Autodesk Inventor part; units mm, degrees
(part 2 of 3)
  arc A299 (127, -169.8625) -> (130.175, -173.0375) centre (130.175, -169.8625) ccw
  arc A300 (132.08, -138.7475) -> (127, -141.2875) centre (130.175, -141.2875) ccw
  arc A301 (136.525, -119.0625) -> (134.62, -124.7775) centre (136.525, -122.2375) ccw
  line L312 (172.72, -153.3525) -> (134.62, -124.7775)
  line L313 (136.525, -119.0625) -> (174.625, -119.0625)
  line L314 (177.8, -122.2375) -> (177.8, -150.8125)
  line L315 (170.18, -167.3225) -> (132.08, -138.7475)
  line L316 (130.175, -173.0375) -> (168.275, -173.0375)
  arc A302 (168.275, -173.0375) -> (170.18, -167.3225) centre (168.275, -169.8625) ccw
  line L317 (-187.4223, -179.3875) -> (-42.9584, -179.3875) construction
  line L318 (-189.0098, -179.3875) -> (-44.5459, -179.3875) construction
  arc A303 (106.68, -124.7775) -> (104.775, -119.0625) centre (104.775, -122.2375) ccw
  line L319 (63.5, -122.2375) -> (63.5, -150.8125)
  arc A304 (63.5, -150.8125) -> (68.58, -153.3525) centre (66.675, -150.8125) ccw
  line L320 (68.58, -153.3525) -> (106.68, -124.7775)
  arc A305 (114.3, -141.2875) -> (109.22, -138.7475) centre (111.125, -141.2875) ccw
  line L321 (71.12, -167.3225) -> (109.22, -138.7475)
  line L322 (111.125, -173.0375) -> (73.025, -173.0375)
  line L323 (120.65, 393.4968) -> (120.65, 317.2968) construction
  line L324 (114.3, -141.2875) -> (114.3, -169.8625)
  arc A306 (111.125, -173.0375) -> (114.3, -169.8625) centre (111.125, -169.8625) ccw
  arc A307 (114.3, -188.9125) -> (111.125, -185.7375) centre (111.125, -188.9125) ccw
  line L325 (114.3, -217.4875) -> (114.3, -188.9125)
  line L326 (111.125, -185.7375) -> (73.025, -185.7375)
  arc A308 (73.025, -185.7375) -> (71.12, -191.4525) centre (73.025, -188.9125) ccw
  line L327 (71.12, -191.4525) -> (109.22, -220.0275)
  arc A309 (68.58, -205.4225) -> (63.5, -207.9625) centre (66.675, -207.9625) ccw
  line L328 (68.58, -205.4225) -> (106.68, -233.9975)
  line L329 (104.775, -239.7125) -> (66.675, -239.7125)
  line L330 (63.5, -236.5375) -> (63.5, -207.9625)
  arc A310 (63.5, -236.5375) -> (66.675, -239.7125) centre (66.675, -236.5375) ccw
  arc A311 (71.12, -167.3225) -> (73.025, -173.0375) centre (73.025, -169.8625) ccw
  line L331 (127, -217.4875) -> (127, -188.9125)
  arc A312 (104.775, -239.7125) -> (106.68, -233.9975) centre (104.775, -236.5375) ccw
  arc A313 (109.22, -220.0275) -> (114.3, -217.4875) centre (111.125, -217.4875) ccw
  arc A314 (177.8, -122.2375) -> (174.625, -119.0625) centre (174.625, -122.2375) ccw
  arc A315 (172.72, -153.3525) -> (177.8, -150.8125) centre (174.625, -150.8125) ccw
  arc A316 (198.12, -167.3225) -> (200.025, -173.0375) centre (200.025, -169.8625) ccw
  arc A317 (190.5, -150.8125) -> (195.58, -153.3525) centre (193.675, -150.8125) ccw
  line L332 (190.5, -122.2375) -> (190.5, -150.8125)
  arc A318 (193.675, -119.0625) -> (190.5, -122.2375) centre (193.675, -122.2375) ccw
  arc A319 (130.175, -185.7375) -> (127, -188.9125) centre (130.175, -188.9125) ccw
  arc A320 (127, -217.4875) -> (132.08, -220.0275) centre (130.175, -217.4875) ccw
  line L333 (130.175, -185.7375) -> (168.275, -185.7375)
  line L334 (177.8, -236.5375) -> (177.8, -207.9625)
  arc A321 (170.18, -191.4525) -> (168.275, -185.7375) centre (168.275, -188.9125) ccw
  line L335 (195.58, -153.3525) -> (233.68, -124.7775)
  line L336 (231.775, -119.0625) -> (193.675, -119.0625)
  arc A322 (241.3, -141.2875) -> (236.22, -138.7475) centre (238.125, -141.2875) ccw
  line L337 (198.12, -167.3225) -> (236.22, -138.7475)
  arc A323 (241.3, -188.9125) -> (238.125, -185.7375) centre (238.125, -188.9125) ccw
  arc A324 (238.125, -173.0375) -> (241.3, -169.8625) centre (238.125, -169.8625) ccw
  arc A325 (236.22, -220.0275) -> (241.3, -217.4875) centre (238.125, -217.4875) ccw
  arc A326 (231.775, -239.7125) -> (233.68, -233.9975) centre (231.775, -236.5375) ccw
  line L338 (170.18, -191.4525) -> (132.08, -220.0275)
  arc A327 (177.8, -207.9625) -> (172.72, -205.4225) centre (174.625, -207.9625) ccw
  arc A328 (174.625, -239.7125) -> (177.8, -236.5375) centre (174.625, -236.5375) ccw
  line L339 (136.525, -239.7125) -> (174.625, -239.7125)
  arc A329 (134.62, -233.9975) -> (136.525, -239.7125) centre (136.525, -236.5375) ccw
  line L340 (172.72, -205.4225) -> (134.62, -233.9975)
  line L341 (241.3, -141.2875) -> (241.3, -169.8625)
  arc A330 (233.68, -124.7775) -> (231.775, -119.0625) centre (231.775, -122.2375) ccw
  line L342 (238.125, -173.0375) -> (200.025, -173.0375)
  line L343 (241.3, -217.4875) -> (241.3, -188.9125)
  line L344 (238.125, -185.7375) -> (200.025, -185.7375)
  arc A331 (200.025, -185.7375) -> (198.12, -191.4525) centre (200.025, -188.9125) ccw
  line L345 (198.12, -191.4525) -> (236.22, -220.0275)
  arc A332 (195.58, -205.4225) -> (190.5, -207.9625) centre (193.675, -207.9625) ccw
  line L346 (195.58, -205.4225) -> (233.68, -233.9975)
  line L347 (231.775, -239.7125) -> (193.675, -239.7125)
  line L348 (190.5, -236.5375) -> (190.5, -207.9625)
  arc A333 (190.5, -236.5375) -> (193.675, -239.7125) centre (193.675, -236.5375) ccw
  arc A334 (168.275, -306.3875) -> (170.18, -300.6725) centre (168.275, -303.2125) ccw
  line L349 (127, -274.6375) -> (127, -303.2125)
  line L350 (120.65, 395.0843) -> (120.65, 318.8843) construction
  line L351 (170.18, -300.6725) -> (132.08, -272.0975)
  arc A335 (132.08, -272.0975) -> (127, -274.6375) centre (130.175, -274.6375) ccw
  arc A336 (172.72, -286.7025) -> (177.8, -284.1625) centre (174.625, -284.1625) ccw
  line L352 (172.72, -286.7025) -> (134.62, -258.1275)
  line L353 (136.525, -252.4125) -> (174.625, -252.4125)
  line L354 (177.8, -255.5875) -> (177.8, -284.1625)
  arc A337 (177.8, -255.5875) -> (174.625, -252.4125) centre (174.625, -255.5875) ccw
  arc A338 (231.775, -373.0625) -> (233.68, -367.3475) centre (231.775, -369.8875) ccw
  arc A339 (45.72, -286.7025) -> (50.8, -284.1625) centre (47.625, -284.1625) ccw
  arc A340 (50.8, -255.5875) -> (47.625, -252.4125) centre (47.625, -255.5875) ccw
  arc A341 (66.675, -252.4125) -> (63.5, -255.5875) centre (66.675, -255.5875) ccw
  line L355 (63.5, -255.5875) -> (63.5, -284.1625)
  arc A342 (63.5, -284.1625) -> (68.58, -286.7025) centre (66.675, -284.1625) ccw
  line L356 (50.8, -255.5875) -> (50.8, -284.1625)
  line L357 (63.5, -369.8875) -> (63.5, -341.3125)
  arc A343 (63.5, -369.8875) -> (66.675, -373.0625) centre (66.675, -369.8875) ccw
  arc A344 (68.58, -338.7725) -> (63.5, -341.3125) centre (66.675, -341.3125) ccw
  line L358 (104.775, -373.0625) -> (66.675, -373.0625)
  line L359 (68.58, -338.7725) -> (106.68, -367.3475)
  line L360 (71.12, -324.8025) -> (109.22, -353.3775)
  arc A345 (71.12, -300.6725) -> (73.025, -306.3875) centre (73.025, -303.2125) ccw
  arc A346 (73.025, -319.0875) -> (71.12, -324.8025) centre (73.025, -322.2625) ccw
  line L361 (111.125, -306.3875) -> (73.025, -306.3875)
  line L362 (111.125, -319.0875) -> (73.025, -319.0875)
  arc A347 (111.125, -306.3875) -> (114.3, -303.2125) centre (111.125, -303.2125) ccw
  line L363 (104.775, -252.4125) -> (66.675, -252.4125)
  arc A348 (106.68, -258.1275) -> (104.775, -252.4125) centre (104.775, -255.5875) ccw
  line L364 (68.58, -286.7025) -> (106.68, -258.1275)
  line L365 (71.12, -300.6725) -> (109.22, -272.0975)
  arc A349 (114.3, -274.6375) -> (109.22, -272.0975) centre (111.125, -274.6375) ccw
  line L366 (114.3, -274.6375) -> (114.3, -303.2125)
  arc A350 (130.175, -319.0875) -> (127, -322.2625) centre (130.175, -322.2625) ccw
  line L367 (114.3, -350.8375) -> (114.3, -322.2625)
  arc A351 (104.775, -373.0625) -> (106.68, -367.3475) centre (104.775, -369.8875) ccw
  arc A352 (109.22, -353.3775) -> (114.3, -350.8375) centre (111.125, -350.8375) ccw
  line L368 (127, -350.8375) -> (127, -322.2625)
  arc A353 (127, -350.8375) -> (132.08, -353.3775) centre (130.175, -350.8375) ccw
  arc A354 (134.62, -367.3475) -> (136.525, -373.0625) centre (136.525, -369.8875) ccw
  arc A355 (136.525, -252.4125) -> (134.62, -258.1275) centre (136.525, -255.5875) ccw
  arc A356 (170.18, -324.8025) -> (168.275, -319.0875) centre (168.275, -322.2625) ccw
  arc A357 (127, -303.2125) -> (130.175, -306.3875) centre (130.175, -303.2125) ccw
  line L369 (130.175, -319.0875) -> (168.275, -319.0875)
  line L370 (130.175, -306.3875) -> (168.275, -306.3875)
  line L371 (170.18, -324.8025) -> (132.08, -353.3775)
  line L372 (172.72, -338.7725) -> (134.62, -367.3475)
  line L373 (136.525, -373.0625) -> (174.625, -373.0625)
  arc A358 (174.625, -373.0625) -> (177.8, -369.8875) centre (174.625, -369.8875) ccw
  arc A359 (177.8, -341.3125) -> (172.72, -338.7725) centre (174.625, -341.3125) ccw
  line L374 (190.5, -369.8875) -> (190.5, -341.3125)
  line L375 (177.8, -369.8875) -> (177.8, -341.3125)
  arc A360 (190.5, -369.8875) -> (193.675, -373.0625) centre (193.675, -369.8875) ccw
  arc A361 (198.12, -300.6725) -> (200.025, -306.3875) centre (200.025, -303.2125) ccw
  arc A362 (241.3, -274.6375) -> (236.22, -272.0975) centre (238.125, -274.6375) ccw
  line L376 (238.125, -306.3875) -> (200.025, -306.3875)
  line L377 (198.12, -300.6725) -> (236.22, -272.0975)
  arc A363 (233.68, -258.1275) -> (231.775, -252.4125) centre (231.775, -255.5875) ccw
  arc A364 (190.5, -284.1625) -> (195.58, -286.7025) centre (193.675, -284.1625) ccw
  line L378 (195.58, -286.7025) -> (233.68, -258.1275)
  line L379 (231.775, -252.4125) -> (193.675, -252.4125)
  arc A365 (193.675, -252.4125) -> (190.5, -255.5875) centre (193.675, -255.5875) ccw
  line L380 (190.5, -255.5875) -> (190.5, -284.1625)
  line L381 (241.3, -274.6375) -> (241.3, -303.2125)
  arc A366 (238.125, -306.3875) -> (241.3, -303.2125) centre (238.125, -303.2125) ccw
  arc A367 (241.3, -322.2625) -> (238.125, -319.0875) centre (238.125, -322.2625) ccw
  arc A368 (200.025, -319.0875) -> (198.12, -324.8025) centre (200.025, -322.2625) ccw
  line L382 (238.125, -319.0875) -> (200.025, -319.0875)
  arc A369 (236.22, -353.3775) -> (241.3, -350.8375) centre (238.125, -350.8375) ccw
  line L383 (231.775, -373.0625) -> (193.675, -373.0625)
  line L384 (195.58, -338.7725) -> (233.68, -367.3475)
  line L385 (241.3, -350.8375) -> (241.3, -322.2625)
  line L386 (198.12, -324.8025) -> (236.22, -353.3775)
  arc A370 (195.58, -338.7725) -> (190.5, -341.3125) centre (193.675, -341.3125) ccw
  arc A371 (114.3, -322.2625) -> (111.125, -319.0875) centre (111.125, -322.2625) ccw
  line L387 (-142.875, -306.3875) -> (-180.975, -306.3875)
  line L388 (-123.825, -306.3875) -> (-85.725, -306.3875)
  arc A372 (-142.875, -306.3875) -> (-139.7, -303.2125) centre (-142.875, -303.2125) ccw
  line L389 (-185.8348, -312.7375) -> (-41.3709, -312.7375) construction
  line L390 (-189.0098, -312.7375) -> (-44.5459, -312.7375) construction
  line L391 (-127, -350.8375) -> (-127, -322.2625)
  arc A373 (-139.7, -322.2625) -> (-142.875, -319.0875) centre (-142.875, -322.2625) ccw
  line L392 (-187.4223, -312.7375) -> (-42.9584, -312.7375) construction
  line L393 (-187.4223, -312.7375) -> (-42.9584, -312.7375) construction
  arc A374 (-190.5, -369.8875) -> (-187.325, -373.0625) centre (-187.325, -369.8875) ccw
  arc A375 (-117.475, -252.4125) -> (-119.38, -258.1275) centre (-117.475, -255.5875) ccw
  line L394 (-83.82, -300.6725) -> (-121.92, -272.0975)
  line L395 (-81.28, -286.7025) -> (-119.38, -258.1275)
  line L396 (-117.475, -252.4125) -> (-79.375, -252.4125)
  arc A376 (-76.2, -255.5875) -> (-79.375, -252.4125) centre (-79.375, -255.5875) ccw
  line L397 (-76.2, -255.5875) -> (-76.2, -284.1625)
  line L398 (-142.875, -319.0875) -> (-180.975, -319.0875)
  line L399 (-182.88, -324.8025) -> (-144.78, -353.3775)
  arc A377 (-180.975, -319.0875) -> (-182.88, -324.8025) centre (-180.975, -322.2625) ccw
  line L400 (-185.42, -338.7725) -> (-147.32, -367.3475)
  line L401 (-149.225, -373.0625) -> (-187.325, -373.0625)
  line L402 (-190.5, -369.8875) -> (-190.5, -341.3125)
  arc A378 (-185.42, -338.7725) -> (-190.5, -341.3125) centre (-187.325, -341.3125) ccw
  arc A379 (-127, -303.2125) -> (-123.825, -306.3875) centre (-123.825, -303.2125) ccw
  line L403 (-190.5, -255.5875) -> (-190.5, -284.1625)
  arc A380 (-187.325, -252.4125) -> (-190.5, -255.5875) centre (-187.325, -255.5875) ccw
  arc A381 (-190.5, -284.1625) -> (-185.42, -286.7025) centre (-187.325, -284.1625) ccw
  arc A382 (-182.88, -300.6725) -> (-180.975, -306.3875) centre (-180.975, -303.2125) ccw
  line L404 (-149.225, -252.4125) -> (-187.325, -252.4125)
  line L405 (-185.42, -286.7025) -> (-147.32, -258.1275)
  line L406 (-182.88, -300.6725) -> (-144.78, -272.0975)
  line L407 (-139.7, -350.8375) -> (-139.7, -322.2625)
  line L408 (3.175, -306.3875) -> (41.275, -306.3875)
  arc A383 (41.275, -306.3875) -> (43.18, -300.6725) centre (41.275, -303.2125) ccw
  line L409 (43.18, -300.6725) -> (5.08, -272.0975)
  line L410 (45.72, -286.7025) -> (7.62, -258.1275)
  line L411 (9.525, -252.4125) -> (47.625, -252.4125)
  arc A384 (9.525, -252.4125) -> (7.62, -258.1275) centre (9.525, -255.5875) ccw
  line L412 (0, -350.8375) -> (0, -322.2625)
  arc A385 (0, -350.8375) -> (5.08, -353.3775) centre (3.175, -350.8375) ccw
  line L413 (3.175, -319.0875) -> (41.275, -319.0875)
  arc A386 (43.18, -324.8025) -> (41.275, -319.0875) centre (41.275, -322.2625) ccw
  line L414 (43.18, -324.8025) -> (5.08, -353.3775)
  arc A387 (7.62, -367.3475) -> (9.525, -373.0625) centre (9.525, -369.8875) ccw
  arc A388 (50.8, -341.3125) -> (45.72, -338.7725) centre (47.625, -341.3125) ccw
  line L415 (45.72, -338.7725) -> (7.62, -367.3475)
  line L416 (50.8, -369.8875) -> (50.8, -341.3125)
  line L417 (9.525, -373.0625) -> (47.625, -373.0625)
  arc A389 (47.625, -373.0625) -> (50.8, -369.8875) centre (47.625, -369.8875) ccw
  arc A390 (3.175, -319.0875) -> (0, -322.2625) centre (3.175, -322.2625) ccw
  line L418 (0, -274.6375) -> (0, -303.2125)
  arc A391 (5.08, -272.0975) -> (0, -274.6375) centre (3.175, -274.6375) ccw
  arc A392 (0, -303.2125) -> (3.175, -306.3875) centre (3.175, -303.2125) ccw
  line L419 (-63.5, -255.5875) -> (-63.5, -284.1625)
  arc A393 (-60.325, -252.4125) -> (-63.5, -255.5875) centre (-60.325, -255.5875) ccw
  arc A394 (-15.875, -306.3875) -> (-12.7, -303.2125) centre (-15.875, -303.2125) ccw
  line L420 (-12.7, -274.6375) -> (-12.7, -303.2125)
  arc A395 (-12.7, -274.6375) -> (-17.78, -272.0975) centre (-15.875, -274.6375) ccw
  line L421 (-15.875, -319.0875) -> (-53.975, -319.0875)
  line L422 (-6.35, 395.0843) -> (-6.35, 318.8843) construction
  line L423 (-15.875, -306.3875) -> (-53.975, -306.3875)
  line L424 (-55.88, -300.6725) -> (-17.78, -272.0975)
  arc A396 (-20.32, -258.1275) -> (-22.225, -252.4125) centre (-22.225, -255.5875) ccw
  line L425 (-58.42, -286.7025) -> (-20.32, -258.1275)
  line L426 (-22.225, -252.4125) -> (-60.325, -252.4125)
  line L427 (-12.7, -350.8375) -> (-12.7, -322.2625)
  arc A397 (-53.975, -319.0875) -> (-55.88, -324.8025) centre (-53.975, -322.2625) ccw
  arc A398 (-63.5, -369.8875) -> (-60.325, -373.0625) centre (-60.325, -369.8875) ccw
  line L428 (-22.225, -373.0625) -> (-60.325, -373.0625)
  line L429 (-58.42, -338.7725) -> (-20.32, -367.3475)
  line L430 (-55.88, -324.8025) -> (-17.78, -353.3775)
  arc A399 (-22.225, -373.0625) -> (-20.32, -367.3475) centre (-22.225, -369.8875) ccw
  arc A400 (-17.78, -353.3775) -> (-12.7, -350.8375) centre (-15.875, -350.8375) ccw
  arc A401 (-12.7, -322.2625) -> (-15.875, -319.0875) centre (-15.875, -322.2625) ccw
  arc A402 (-79.375, -373.0625) -> (-76.2, -369.8875) centre (-79.375, -369.8875) ccw
  arc A403 (-83.82, -324.8025) -> (-85.725, -319.0875) centre (-85.725, -322.2625) ccw
  arc A404 (-76.2, -341.3125) -> (-81.28, -338.7725) centre (-79.375, -341.3125) ccw
  line L431 (-63.5, -369.8875) -> (-63.5, -341.3125)
  arc A405 (-58.42, -338.7725) -> (-63.5, -341.3125) centre (-60.325, -341.3125) ccw
  line L432 (-139.7, -274.6375) -> (-139.7, -303.2125)
  arc A406 (-121.92, -272.0975) -> (-127, -274.6375) centre (-123.825, -274.6375) ccw
  line L433 (-127, -274.6375) -> (-127, -303.2125)
  line L434 (-133.35, 393.4968) -> (-133.35, 317.2968) construction
  arc A407 (-139.7, -274.6375) -> (-144.78, -272.0975) centre (-142.875, -274.6375) ccw
  arc A408 (-147.32, -258.1275) -> (-149.225, -252.4125) centre (-149.225, -255.5875) ccw
  arc A409 (-123.825, -319.0875) -> (-127, -322.2625) centre (-123.825, -322.2625) ccw
  arc A410 (-127, -350.8375) -> (-121.92, -353.3775) centre (-123.825, -350.8375) ccw
  arc A411 (-119.38, -367.3475) -> (-117.475, -373.0625) centre (-117.475, -369.8875) ccw
  line L435 (-123.825, -319.0875) -> (-85.725, -319.0875)
  line L436 (-83.82, -324.8025) -> (-121.92, -353.3775)
  line L437 (-81.28, -338.7725) -> (-119.38, -367.3475)
  line L438 (-76.2, -369.8875) -> (-76.2, -341.3125)
  line L439 (-117.475, -373.0625) -> (-79.375, -373.0625)
  arc A412 (-149.225, -373.0625) -> (-147.32, -367.3475) centre (-149.225, -369.8875) ccw
  arc A413 (-144.78, -353.3775) -> (-139.7, -350.8375) centre (-142.875, -350.8375) ccw
  arc A414 (-85.725, -306.3875) -> (-83.82, -300.6725) centre (-85.725, -303.2125) ccw
  arc A415 (-81.28, -286.7025) -> (-76.2, -284.1625) centre (-79.375, -284.1625) ccw
  arc A416 (-63.5, -284.1625) -> (-58.42, -286.7025) centre (-60.325, -284.1625) ccw
  arc A417 (-55.88, -300.6725) -> (-53.975, -306.3875) centre (-53.975, -303.2125) ccw
  arc A418 (-182.88, -434.0225) -> (-180.975, -439.7375) centre (-180.975, -436.5625) ccw
  arc A419 (-142.875, -439.7375) -> (-139.7, -436.5625) centre (-142.875, -436.5625) ccw
  line L440 (-190.5, -388.9375) -> (-190.5, -417.5125)
  arc A420 (-187.325, -385.7625) -> (-190.5, -388.9375) centre (-187.325, -388.9375) ccw
  arc A421 (-121.92, -405.4475) -> (-127, -407.9875) centre (-123.825, -407.9875) ccw
  line L441 (-127, -407.9875) -> (-127, -436.5625)
  line L442 (-133.35, 393.4968) -> (-133.35, 317.2968) construction
  line L443 (-130.175, 395.0843) -> (-130.175, 318.8843) construction
  arc A422 (-127, -436.5625) -> (-123.825, -439.7375) centre (-123.825, -436.5625) ccw
  line L444 (-123.825, -439.7375) -> (-85.725, -439.7375)
  arc A423 (-85.725, -439.7375) -> (-83.82, -434.0225) centre (-85.725, -436.5625) ccw
  arc A424 (-55.88, -434.0225) -> (-53.975, -439.7375) centre (-53.975, -436.5625) ccw
  line L445 (-58.42, -420.0525) -> (-20.32, -391.4775)
  line L446 (-63.5, -388.9375) -> (-63.5, -417.5125)
  arc A425 (-63.5, -417.5125) -> (-58.42, -420.0525) centre (-60.325, -417.5125) ccw
  arc A426 (-60.325, -385.7625) -> (-63.5, -388.9375) centre (-60.325, -388.9375) ccw
  arc A427 (-117.475, -385.7625) -> (-119.38, -391.4775) centre (-117.475, -388.9375) ccw
  line L447 (-83.82, -434.0225) -> (-121.92, -405.4475)
  line L448 (-81.28, -420.0525) -> (-119.38, -391.4775)
  arc A428 (-81.28, -420.0525) -> (-76.2, -417.5125) centre (-79.375, -417.5125) ccw
  line L449 (-76.2, -388.9375) -> (-76.2, -417.5125)
  line L450 (-117.475, -385.7625) -> (-79.375, -385.7625)
  arc A429 (-76.2, -388.9375) -> (-79.375, -385.7625) centre (-79.375, -388.9375) ccw
  arc A430 (-190.5, -417.5125) -> (-185.42, -420.0525) centre (-187.325, -417.5125) ccw
  line L451 (-149.225, -385.7625) -> (-187.325, -385.7625)
  arc A431 (-147.32, -391.4775) -> (-149.225, -385.7625) centre (-149.225, -388.9375) ccw
  line L452 (-185.42, -420.0525) -> (-147.32, -391.4775)
  arc A432 (-139.7, -407.9875) -> (-144.78, -405.4475) centre (-142.875, -407.9875) ccw
  line L453 (-182.88, -434.0225) -> (-144.78, -405.4475)
  line L454 (-142.875, -439.7375) -> (-180.975, -439.7375)
  line L455 (-139.7, -407.9875) -> (-139.7, -436.5625)
  line L456 (-22.225, -385.7625) -> (-60.325, -385.7625)
  line L457 (3.175, -439.7375) -> (41.275, -439.7375)
  arc A433 (9.525, -385.7625) -> (7.62, -391.4775) centre (9.525, -388.9375) ccw
  arc A434 (41.275, -439.7375) -> (43.18, -434.0225) centre (41.275, -436.5625) ccw
  line L458 (43.18, -434.0225) -> (5.08, -405.4475)
  arc A435 (45.72, -420.0525) -> (50.8, -417.5125) centre (47.625, -417.5125) ccw
  line L459 (45.72, -420.0525) -> (7.62, -391.4775)
  line L460 (9.525, -385.7625) -> (47.625, -385.7625)
  line L461 (50.8, -388.9375) -> (50.8, -417.5125)
  arc A436 (50.8, -388.9375) -> (47.625, -385.7625) centre (47.625, -388.9375) ccw
  arc A437 (-20.32, -391.4775) -> (-22.225, -385.7625) centre (-22.225, -388.9375) ccw
  arc A438 (-12.7, -407.9875) -> (-17.78, -405.4475) centre (-15.875, -407.9875) ccw
  line L462 (-55.88, -434.0225) -> (-17.78, -405.4475)
  line L463 (-15.875, -439.7375) -> (-53.975, -439.7375)
  line L464 (-6.35, 395.0843) -> (-6.35, 318.8843) construction
  line L465 (-3.175, 396.6718) -> (-3.175, 320.4718) construction
  arc A439 (5.08, -405.4475) -> (0, -407.9875) centre (3.175, -407.9875) ccw
  line L466 (-12.7, -407.9875) -> (-12.7, -436.5625)
  arc A440 (-15.875, -439.7375) -> (-12.7, -436.5625) centre (-15.875, -436.5625) ccw
  arc A441 (0, -436.5625) -> (3.175, -439.7375) centre (3.175, -436.5625) ccw
  line L467 (0, -407.9875) -> (0, -436.5625)
  arc A442 (111.125, -439.7375) -> (114.3, -436.5625) centre (111.125, -436.5625) ccw
  line L468 (114.3, -407.9875) -> (114.3, -436.5625)
  arc A443 (114.3, -407.9875) -> (109.22, -405.4475) centre (111.125, -407.9875) ccw
  line L469 (111.125, -439.7375) -> (73.025, -439.7375)
  line L470 (123.825, 396.6718) -> (123.825, 320.4718) construction
  line L471 (120.65, 395.0843) -> (120.65, 318.8843) construction
  arc A444 (71.12, -434.0225) -> (73.025, -439.7375) centre (73.025, -436.5625) ccw
  line L472 (71.12, -434.0225) -> (109.22, -405.4475)
  arc A445 (63.5, -417.5125) -> (68.58, -420.0525) centre (66.675, -417.5125) ccw
  line L473 (68.58, -420.0525) -> (106.68, -391.4775)
  line L474 (104.775, -385.7625) -> (66.675, -385.7625)
  line L475 (63.5, -388.9375) -> (63.5, -417.5125)
  arc A446 (66.675, -385.7625) -> (63.5, -388.9375) centre (66.675, -388.9375) ccw
  line L476 (130.175, -439.7375) -> (168.275, -439.7375)
  line L477 (127, -407.9875) -> (127, -436.5625)
  arc A447 (127, -436.5625) -> (130.175, -439.7375) centre (130.175, -436.5625) ccw
  arc A448 (132.08, -405.4475) -> (127, -407.9875) centre (130.175, -407.9875) ccw
  arc A449 (136.525, -385.7625) -> (134.62, -391.4775) centre (136.525, -388.9375) ccw
  line L478 (172.72, -420.0525) -> (134.62, -391.4775)
  line L479 (136.525, -385.7625) -> (174.625, -385.7625)
  line L480 (170.18, -434.0225) -> (132.08, -405.4475)
  arc A450 (172.72, -420.0525) -> (177.8, -417.5125) centre (174.625, -417.5125) ccw
  arc A451 (168.275, -439.7375) -> (170.18, -434.0225) centre (168.275, -436.5625) ccw
  arc A452 (106.68, -391.4775) -> (104.775, -385.7625) centre (104.775, -388.9375) ccw
  line L481 (241.3, -407.9875) -> (241.3, -436.5625)
  arc A453 (238.125, -439.7375) -> (241.3, -436.5625) centre (238.125, -436.5625) ccw
  line L482 (177.8, -388.9375) -> (177.8, -417.5125)
  arc A454 (177.8, -388.9375) -> (174.625, -385.7625) centre (174.625, -388.9375) ccw
  arc A455 (198.12, -434.0225) -> (200.025, -439.7375) centre (200.025, -436.5625) ccw
  arc A456 (190.5, -417.5125) -> (195.58, -420.0525) centre (193.675, -417.5125) ccw
  line L483 (190.5, -388.9375) -> (190.5, -417.5125)
  arc A457 (193.675, -385.7625) -> (190.5, -388.9375) centre (193.675, -388.9375) ccw
  line L484 (198.12, -434.0225) -> (236.22, -405.4475)
  arc A458 (241.3, -407.9875) -> (236.22, -405.4475) centre (238.125, -407.9875) ccw
  line L485 (195.58, -420.0525) -> (233.68, -391.4775)
  line L486 (231.775, -385.7625) -> (193.675, -385.7625)
  arc A459 (233.68, -391.4775) -> (231.775, -385.7625) centre (231.775, -388.9375) ccw
  line L487 (238.125, -439.7375) -> (200.025, -439.7375)
  line L488 (-171.45, -101.6) -> (-228.6, -101.6) projected
  line L489 (-228.6, -127) -> (-228.6, -101.6) projected
  line L490 (-330.2, -127) -> (-228.6, -127) projected
  line L491 (-330.2, -203.2) -> (-330.2, -127) projected
  line L492 (-228.6, -203.2) -> (-330.2, -203.2) projected
  line L493 (-228.6, -457.2) -> (-228.6, -203.2) projected
  line L494 (279.4, -457.2) -> (-228.6, -457.2) projected
  line L495 (279.4, -203.2) -> (279.4, -457.2) projected
  line L496 (381, -203.2) -> (279.4, -203.2) projected
  line L497 (381, -127) -> (381, -203.2) projected
  line L498 (279.4, -127) -> (381, -127) projected
  line L499 (279.4, -101.6) -> (279.4, -127) projected
  line L500 (279.4, -101.6) -> (222.25, -101.6) projected
  line L501 (222.25, -101.6) -> (222.25, 50.8) projected
  line L502 (222.25, 50.8) -> (279.4, 50.8) projected
  line L503 (279.4, 76.2) -> (279.4, 50.8) projected
  line L504 (381, 76.2) -> (279.4, 76.2) projected
  line L505 (381, 152.4) -> (381, 76.2) projected
  line L506 (279.4, 152.4) -> (381, 152.4) projected
  line L507 (279.4, 406.4) -> (279.4, 152.4) projected
  line L508 (-228.6, 406.4) -> (279.4, 406.4) projected
  line L509 (-228.6, 152.4) -> (-228.6, 406.4) projected
  line L510 (-330.2, 152.4) -> (-228.6, 152.4) projected
  line L511 (-330.2, 76.2) -> (-330.2, 152.4) projected
  line L512 (-228.6, 76.2) -> (-330.2, 76.2) projected
  line L513 (-228.6, 50.8) -> (-228.6, 76.2) projected
  line L514 (-228.6, 50.8) -> (-171.45, 50.8) projected
  line L515 (-171.45, 50.8) -> (-171.45, -101.6) projected
  circle A460 centre (368.3, 88.9) radius 3.3782 projected
  circle A461 centre (368.3, 114.3) radius 3.3782 projected
  circle A462 centre (368.3, 139.7) radius 3.3782 projected
  circle A463 centre (368.3, -190.5) radius 3.3782 projected
  circle A464 centre (368.3, -165.1) radius 3.3782 projected
  circle A465 centre (368.3, -139.7) radius 3.3782 projected
  circle A466 centre (-317.5, -190.5) radius 3.3782 projected
  circle A467 centre (-317.5, -165.1) radius 3.3782 projected
  circle A468 centre (-317.5, -139.7) radius 3.3782 projected
  circle A469 centre (-317.5, 88.9) radius 3.3782 projected
  circle A470 centre (-317.5, 114.3) radius 3.3782 projected
  circle A471 centre (-317.5, 139.7) radius 3.3782 projected
  circle A472 centre (266.7, -444.5) radius 3.3782 projected
  circle A473 centre (-215.9, -444.5) radius 3.3782 projected
  circle A474 centre (266.7, -419.1) radius 3.3782 projected
  circle A475 centre (-215.9, -419.1) radius 3.3782 projected
  circle A476 centre (266.7, -393.7) radius 3.3782 projected
  circle A477 centre (-215.9, -393.7) radius 3.3782 projected
  circle A478 centre (266.7, -368.3) radius 3.3782 projected
  circle A479 centre (-215.9, -368.3) radius 3.3782 projected
  circle A480 centre (266.7, -342.9) radius 3.3782 projected
  circle A481 centre (-215.9, -342.9) radius 3.3782 projected
  circle A482 centre (266.7, -317.5) radius 3.3782 projected
  circle A483 centre (-215.9, -317.5) radius 3.3782 projected
  circle A484 centre (266.7, -292.1) radius 3.3782 projected
  circle A485 centre (-215.9, -292.1) radius 3.3782 projected
  circle A486 centre (266.7, -266.7) radius 3.3782 projected
  circle A487 centre (-215.9, -266.7) radius 3.3782 projected
  circle A488 centre (266.7, -241.3) radius 3.3782 projected
  circle A489 centre (-215.9, -241.3) radius 3.3782 projected
  circle A490 centre (266.7, -215.9) radius 3.3782 projected
  circle A491 centre (-215.9, -215.9) radius 3.3782 projected
  circle A492 centre (266.7, -190.5) radius 3.3782 projected
  circle A493 centre (-215.9, -190.5) radius 3.3782 projected
  circle A494 centre (266.7, -165.1) radius 3.3782 projected
  circle A495 centre (-215.9, -165.1) radius 3.3782 projected
  circle A496 centre (266.7, -139.7) radius 3.3782 projected
  circle A497 centre (-215.9, -139.7) radius 3.3782 projected
  circle A498 centre (266.7, -114.3) radius 3.3782 projected
  circle A499 centre (-215.9, -114.3) radius 3.3782 projected
  circle A500 centre (266.7, 63.5) radius 3.3782 projected
  circle A501 centre (-215.9, 63.5) radius 3.3782 projected
  circle A502 centre (266.7, 88.9) radius 3.3782 projected
  circle A503 centre (-215.9, 88.9) radius 3.3782 projected
  circle A504 centre (266.7, 114.3) radius 3.3782 projected
  circle A505 centre (-215.9, 114.3) radius 3.3782 projected
  circle A506 centre (266.7, 139.7) radius 3.3782 projected
  circle A507 centre (-215.9, 139.7) radius 3.3782 projected
  circle A508 centre (266.7, 165.1) radius 3.3782 projected
  circle A509 centre (-215.9, 165.1) radius 3.3782 projected
  circle A510 centre (266.7, 190.5) radius 3.3782 projected
  circle A511 centre (-215.9, 190.5) radius 3.3782 projected
  circle A512 centre (266.7, 215.9) radius 3.3782 projected
  circle A513 centre (-215.9, 215.9) radius 3.3782 projected
  circle A514 centre (266.7, 241.3) radius 3.3782 projected
  circle A515 centre (-215.9, 241.3) radius 3.3782 projected
  circle A516 centre (266.7, 266.7) radius 3.3782 projected
  circle A517 centre (-215.9, 266.7) radius 3.3782 projected
  circle A518 centre (266.7, 292.1) radius 3.3782 projected
  circle A519 centre (-215.9, 292.1) radius 3.3782 projected
  circle A520 centre (266.7, 317.5) radius 3.3782 projected
  circle A521 centre (-215.9, 317.5) radius 3.3782 projected
  circle A522 centre (266.7, 342.9) radius 3.3782 projected
  circle A523 centre (-215.9, 342.9) radius 3.3782 projected
  circle A524 centre (266.7, 368.3) radius 3.3782 projected
  circle A525 centre (-215.9, 368.3) radius 3.3782 projected
  circle A526 centre (266.7, 393.7) radius 3.3782 projected
  circle A527 centre (-215.9, 393.7) radius 3.3782 projected
  point P0 (-190.5, 388.9375)
  point P1 (-190.5, 350.8375)
  point P2 (-139.7, 388.9375)
  point P3 (-190.5, 334.9625)
  point P4 (-139.7, 352.425)
  point P5 (-190.5, 371.475)
  point P6 (-76.2, 388.9375)
  point P7 (-76.2, 350.8375)
  point P8 (-127, 388.9375)
  point P9 (-76.2, 334.9625)
  point P10 (-127, 352.425)
  point P11 (-76.2, 371.475)
  point P12 (-190.5, 268.2875)
  point P13 (-190.5, 306.3875)
  point P14 (-139.7, 268.2875)
  point P15 (-190.5, 322.2625)
  point P16 (-139.7, 304.8)
  point P17 (-190.5, 285.75)
  point P18 (-127, 304.8)
  point P19 (-127, 268.2875)
  point P20 (-76.2, 268.2875)
  point P21 (-76.2, 285.75)
  point P22 (-76.2, 306.3875)
  point P23 (-76.2, 322.2625)
  point P24 (-63.5, 388.9375)
  point P25 (-63.5, 350.8375)
  point P26 (-12.7, 388.9375)
  point P27 (-63.5, 334.9625)
  point P28 (-12.7, 352.425)
  point P29 (-63.5, 371.475)
  point P30 (0, 352.425)
  point P31 (0, 388.9375)
  point P32 (50.8, 388.9375)
  point P33 (50.8, 371.475)
  point P34 (50.8, 350.8375)
  point P35 (50.8, 334.9625)
  point P36 (-63.5, 285.75)
  point P37 (-12.7, 304.8)
  point P38 (-63.5, 268.2875)
  point P39 (-12.7, 268.2875)
  point P40 (50.8, 285.75)
  point P41 (-63.5, 306.3875)
  point P42 (-63.5, 322.2625)
  point P43 (0, 304.8)
  point P44 (50.8, 322.2625)
  point P45 (0, 268.2875)
  point P46 (50.8, 306.3875)
  point P47 (50.8, 268.2875)
  point P48 (-98.425, 388.9375)
  point P49 (-41.275, 388.9375)
  point P50 (63.5, 388.9375)
  point P51 (63.5, 350.8375)
  point P52 (114.3, 388.9375)
  point P53 (63.5, 334.9625)
  point P54 (114.3, 352.425)
  point P55 (63.5, 371.475)
  point P56 (127, 352.425)
  point P57 (127, 388.9375)
  point P58 (177.8, 388.9375)
  point P59 (177.8, 371.475)
  point P60 (177.8, 350.8375)
  point P61 (177.8, 334.9625)
  point P62 (63.5, 285.75)
  point P63 (114.3, 304.8)
  point P64 (63.5, 268.2875)
  point P65 (114.3, 268.2875)
  point P66 (177.8, 285.75)
  point P67 (63.5, 306.3875)
  point P68 (63.5, 322.2625)
  point P69 (127, 304.8)
  point P70 (177.8, 322.2625)
  point P71 (127, 268.2875)
  point P72 (177.8, 306.3875)
  point P73 (177.8, 268.2875)
  point P74 (190.5, 388.9375)
  point P75 (190.5, 371.475)
  point P76 (190.5, 350.8375)
  point P77 (241.3, 388.9375)
  point P78 (190.5, 334.9625)
  point P79 (241.3, 352.425)
  point P80 (241.3, 304.8)
  point P81 (241.3, 268.2875)
  point P82 (190.5, 285.75)
  point P83 (190.5, 306.3875)
  point P84 (190.5, 268.2875)
  point P85 (190.5, 322.2625)
  point P86 (155.575, 388.9375)
  point P87 (212.725, 388.9375)
  point P88 (28.575, 388.9375)
  point P89 (85.725, 388.9375)
  point P90 (-190.5, 255.5875)
  point P91 (-190.5, 217.4875)
  point P92 (-139.7, 255.5875)
  point P93 (-190.5, 201.6125)
  point P94 (-139.7, 219.075)
  point P95 (-190.5, 238.125)
  point P96 (-127, 219.075)
  point P97 (-127, 255.5875)
  point P98 (-76.2, 255.5875)
  point P99 (-76.2, 238.125)
  point P100 (-76.2, 217.4875)
  point P101 (-76.2, 201.6125)
  point P102 (-190.5, 152.4)
  point P103 (-139.7, 171.45)
  point P104 (-190.5, 134.9375)
  point P105 (-139.7, 134.9375)
  point P106 (-76.2, 152.4)
  point P107 (-190.5, 173.0375)
  point P108 (-190.5, 188.9125)
  point P109 (-127, 171.45)
  point P110 (-76.2, 188.9125)
  point P111 (-127, 134.9375)
  point P112 (-76.2, 173.0375)
  point P113 (-76.2, 134.9375)
  point P114 (-63.5, 255.5875)
  point P115 (-63.5, 238.125)
  point P116 (-63.5, 217.4875)
  point P117 (-12.7, 255.5875)
  point P118 (-63.5, 201.6125)
  point P119 (-12.7, 219.075)
  point P120 (50.8, 134.9375)
  point P121 (50.8, 188.9125)
  point P122 (-12.7, 171.45)
  point P123 (0, 171.45)
  point P124 (50.8, 201.6125)
  point P125 (50.8, 173.0375)
  point P126 (50.8, 152.4)
  point P127 (0, 134.9375)
  point P128 (0, 219.075)
  point P129 (0, 255.5875)
  point P130 (50.8, 255.5875)
  point P131 (50.8, 217.4875)
  point P132 (50.8, 238.125)
  point P133 (-12.7, 134.9375)
  point P134 (-63.5, 152.4)
  point P135 (-63.5, 173.0375)
  point P136 (-63.5, 134.9375)
  point P137 (-63.5, 188.9125)
  point P138 (-98.425, 255.5875)
  point P139 (-41.275, 255.5875)
  point P140 (63.5, 238.125)
  point P141 (63.5, 255.5875)
  point P142 (114.3, 255.5875)
  point P143 (127, 219.075)
  point P144 (127, 255.5875)
  point P145 (177.8, 217.4875)
  point P146 (177.8, 255.5875)
  point P147 (155.575, 255.5875)
  point P148 (177.8, 238.125)
  point P149 (177.8, 201.6125)
  point P150 (63.5, 217.4875)
  point P151 (63.5, 201.6125)
  point P152 (114.3, 219.075)
  point P153 (114.3, 171.45)
  point P154 (63.5, 188.9125)
  point P155 (63.5, 173.0375)
  point P156 (114.3, 134.9375)
  point P157 (63.5, 134.9375)
  point P158 (63.5, 152.4)
  point P159 (127, 171.45)
  point P160 (190.5, 201.6125)
  point P161 (190.5, 217.4875)
  point P162 (190.5, 238.125)
  point P163 (190.5, 255.5875)
  point P164 (212.725, 255.5875)
  point P165 (177.8, 188.9125)
  point P166 (177.8, 152.4)
  point P167 (177.8, 173.0375)
  point P168 (177.8, 134.9375)
  point P169 (241.3, 255.5875)
  point P170 (241.3, 219.075)
  point P171 (241.3, 171.45)
  point P172 (241.3, 134.9375)
  point P173 (190.5, 173.0375)
  point P174 (127, 134.9375)
  point P175 (190.5, 188.9125)
  point P176 (190.5, 152.4)
  point P177 (190.5, 134.9375)
  point P178 (28.575, 255.5875)
  point P179 (85.725, 255.5875)
  point P180 (-190.5, 285.75)
  point P181 (-190.5, 122.2375)
  point P182 (-190.5, 84.1375)
  point P183 (-139.7, 122.2375)
  point P184 (-190.5, 68.2625)
  point P185 (-139.7, 85.725)
  point P186 (-190.5, 104.775)
  point P187 (-127, 85.725)
  point P188 (-127, 122.2375)
  point P189 (-76.2, 122.2375)
  point P190 (-76.2, 104.775)
  point P191 (-76.2, 84.1375)
  point P192 (-76.2, 68.2625)
  point P193 (-63.5, 122.2375)
  point P194 (-63.5, 104.775)
  point P195 (-63.5, 84.1375)
  point P196 (-12.7, 122.2375)
  point P197 (-63.5, 68.2625)
  point P198 (-12.7, 85.725)
  point P199 (50.8, 68.2625)
  dimension "d181" = 50.8
  dimension "d182" = 38.1
  dimension "d184" = 12.7
  dimension "d185" = 3.175
  dimension "d186" = 6.35
  dimension "d187" = 6.35
  dimension "d188" = 38.1
  dimension "d189" = 17.4625
  dimension "d190" = 50.8
  dimension "d191" = 38.1
  dimension "d192" = 12.7
  dimension "d193" = 3.175
  dimension "d194" = 6.35
  dimension "d195" = 6.35
  dimension "d196" = 12.7
  dimension "d197" = 50.8
  dimension "d198" = 38.1
  dimension "d199" = 12.7
  dimension "d200" = 3.175
  dimension "d201" = 6.35
  dimension "d202" = 6.35
  dimension "d203" = 50.8
  dimension "d204" = 38.1
  dimension "d205" = 12.7
  dimension "d206" = 3.175
  dimension "d207" = 12.7
  dimension "d208" = 12.7
  dimension "d209" = 12.7
  dimension "d210" = 38.1
  dimension "d211" = 50.8
  dimension "d212" = 38.1
  dimension "d213" = 12.7
  dimension "d214" = 3.175
  dimension "d215" = 6.35
  dimension "d216" = 6.35
  dimension "d217" = 50.8
  dimension "d218" = 38.1
  dimension "d219" = 12.7
  dimension "d220" = 3.175
  dimension "d221" = 6.35
  dimension "d222" = 6.35
  dimension "d223" = 12.7
  dimension "d224" = 50.8
  dimension "d225" = 38.1
  dimension "d226" = 12.7
  dimension "d227" = 3.175
  dimension "d228" = 6.35
  dimension "d229" = 6.35
  dimension "d230" = 50.8
  dimension "d231" = 38.1
  dimension "d232" = 12.7
  dimension "d233" = 3.175
  dimension "d234" = 12.7
  dimension "d235" = 12.7
  dimension "d236" = 12.7
  dimension "d237" = 12.7
  dimension "d238" = 50.8
  dimension "d239" = 38.1
  dimension "d240" = 12.7
  dimension "d241" = 3.175
  dimension "d242" = 6.35
  dimension "d244" = 50.8
  dimension "d245" = 38.1
  dimension "d246" = 12.7
  constraints: 1104 symmetric about line, 920 end point, 840 point on circle, 560 point on line, 420 centre point, 288 tangent, 120 equal radius, 90 perpendicular, 88 midpoint, 53 vertical alignment, 37 parallel, 18 horizontal alignment, 276 other
  measures "d181" distance of point (-139.7, 388.938) point (-190.5, 388.938)
  measures "d182" distance of point (-190.5, 388.938) point (-190.5, 350.838)
  measures "d184" distance between parallel lines of L29 L27
  measures "d185" radius of A40
  measures "d186" distance between parallel lines of L32 L30
  measures "d187" distance between parallel lines of L38 L39
  measures "d188" distance between parallel lines of L20 L26
  measures "d189" distance between parallel lines of L19 L28
  measures "d190" distance of point (-12.7, 388.938) point (-63.5, 388.938)
  measures "d191" distance of point (-63.5, 388.938) point (-63.5, 350.837)
  measures "d192" distance between parallel lines of L55 L53
  measures "d193" radius of A64
  measures "d194" distance between parallel lines of L58 L56
  measures "d195" distance between parallel lines of L64 L65
  measures "d196" distance between parallel lines of L33 L52
  measures "d197" distance of point (114.3, 388.938) point (63.5, 388.938)
  measures "d198" distance of point (63.5, 388.938) point (63.5, 350.837)
  measures "d199" distance between parallel lines of L81 L79
  measures "d200" radius of A88
  measures "d201" distance between parallel lines of L84 L82
  measures "d202" distance between parallel lines of L90 L91
  measures "d203" distance of point (241.3, 388.938) point (190.5, 388.938)
  measures "d204" distance of point (190.5, 388.938) point (190.5, 350.837)
  measures "d205" distance between parallel lines of L107 L105
  measures "d206" radius of A115
  measures "d207" distance between parallel lines of L86 L104
  measures "d208" distance between parallel lines of L109 L116
  measures "d209" distance between parallel lines of L60 L78
  measures "d210" distance between parallel lines of L18 L108
  measures "d211" distance of point (-139.7, 255.588) point (-190.5, 255.588)
  measures "d212" distance of point (-190.5, 255.588) point (-190.5, 217.488)
  measures "d213" distance between parallel lines of L120 L118
  measures "d214" radius of A124
  measures "d215" distance between parallel lines of L123 L121
  measures "d216" distance between parallel lines of L129 L130
  measures "d217" distance of point (-12.7, 255.588) point (-63.5, 255.588)
  measures "d218" distance of point (-63.5, 255.588) point (-63.5, 217.488)
  measures "d219" distance between parallel lines of L146 L144
  measures "d220" radius of A151
  measures "d221" distance between parallel lines of L159 L147
  measures "d222" distance between parallel lines of L152 L150
  measures "d223" distance between parallel lines of L125 L143
  measures "d224" distance of point (114.3, 255.588) point (63.5, 255.588)
  measures "d225" distance of point (63.5, 255.588) point (63.5, 217.488)
  measures "d226" distance between parallel lines of L180 L179
  measures "d227" radius of A178
  measures "d228" distance between parallel lines of L182 L183
  measures "d229" distance between parallel lines of L175 L177
  measures "d230" distance of point (241.3, 255.588) point (190.5, 255.588)
  measures "d231" distance of point (190.5, 255.588) point (190.5, 217.488)
  measures "d232" distance between parallel lines of L196 L194
  measures "d233" radius of A191
  measures "d234" distance between parallel lines of L173 L191
  measures "d235" distance between parallel lines of L201 L203
  measures "d236" distance between parallel lines of L163 L178
  measures "d237" distance between parallel lines of L48 L126
  measures "d238" distance of point (-139.7, 122.238) point (-190.5, 122.238)
  measures "d239" distance of point (-190.5, 122.238) point (-190.5, 84.138)
  measures "d240" distance between parallel lines of L211 L209
  measures "d241" radius of A208
  measures "d242" distance between parallel lines of L214 L212
  measures "d244" distance of point (-12.7, 122.238) point (-63.5, 122.238)
  measures "d245" distance of point (-63.5, 122.238) point (-63.5, 84.138)
  measures "d246" distance between parallel lines of L224 L222
extrude "Extrusion4" cut sketch "Sketch6" against normal through all keep common part